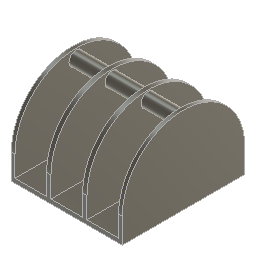
Настольный держатель маленьких кусачек и плоскогубцев(3) (Autodesk Fusion 360 design; units mm, degrees)
Autodesk Fusion 360 part; units mm, degrees
sketch "Sketch1" plane through (0, 0, 0) normal (0, 0, 1) x (1, 0, 0)
  line L0 (11, -40) -> (-11, -40)
  line L1 (-11, -42.5) -> (-11, 42.5)
  line L2 (-11, 40) -> (11, 40)
  line L3 (11, 42.5) -> (11, -42.5)
  line L4 (-13.5, -42.5) -> (-13.5, 42.5)
  line L5 (-13.5, 42.5) -> (13.5, 42.5)
  line L6 (13.5, 42.5) -> (13.5, -42.5)
  line L7 (13.5, -42.5) -> (-13.5, -42.5)
  dimension "d1" = 22
  dimension "d2" = 80
  constraint horizontal L0
  constraint perpendicular L0 L1
  constraint parallel L0 L2
  constraint parallel L1 L3
  constraint coincident L5 L1.end
  constraint coincident L2.start L1
  constraint coincident L5 L3.start
  constraint coincident L2.end L3
  constraint coincident L7 L3.end
  constraint coincident L0.start L3
  constraint coincident L7 L1.start
  constraint coincident L0.end L1
  measures "d1" distance of L2.start L2.end
  measures "d2" distance of L0.end L2.start
extrude "Extrude1" add sketch "Sketch1" along normal blind 3 makes body 1
extrude "Extrude2" add sketch "Sketch1" along normal blind 60 contours L3 L5 L6 L7 | L1 L4 L5 L7 bodies 1
fillet "Fillet1" radius 42.5 4 edges at (12.25, -42.5, 60) (-12.25, -42.5, 60) (12.25, 42.5, 60) (-12.25, 42.5, 60) on bodies 1
sketch "Sketch2" plane through (13.5, 0, 0) normal (1, 0, 0) x (0, 1, 0)
  arc A0 (42.5, 17.5) -> (-42.5, 17.5) centre (0, 17.5) ccw
  line L0 (-42.5, 17.5) -> (-42.5, 0)
  line L1 (-42.5, 0) -> (42.5, 0)
  line L2 (42.5, 0) -> (42.5, 17.5)
  circle A1 centre (0, 54) radius 5
  dimension "d10" = 10
  measures "d10" diameter of A1
extrude "Extrude3" add sketch "Sketch2" against normal blind 27 contours A1 bodies 1
pattern_linear "R-Pattern1" count 3 spacing 25 along (1, 0, 0) of bodies 1 makes body 2 at (38.5, 0.0028, 31.6723) makes body 3 at (63.5, 0.0028, 31.6723)
combine "Combine1" operation add target body 1 tool bodies 2 3
